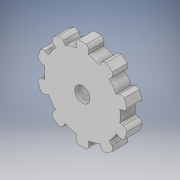
# Autodesk Inventor part: 10 ul Middle Gear
Saved by Autodesk Inventor 2017 (Build 210142000, 142)
## iProperties
Created: 2018-03-09
Part Number: 10 ul Middle Gear
Material: Generic
Document SubType Name: Modeling
Designer: Russ
Density: 1 g/cm^3
Appearance: Default
Author: Russ
Autodesk Inventor part; units mm, degrees
ref_plane "YZ Plane" through (0, 0, 0) normal (1, 0, 0) x (0, 1, 0)
ref_plane "XZ Plane" through (0, 0, 0) normal (0, 1, 0) x (-1, 0, 0)
ref_plane "XY Plane" through (0, 0, 0) normal (0, 0, 1) x (1, 0, 0)
sketch "Sketch1" plane through (0, 0, 0) normal (0, 0, 1) x (1, 0, 0)
  arc A0 (-1.49, 9.4077) -> (1.49, 9.4077) centre (0, 0) ccw
  line L0 (0, 9.525) -> (0, 11.43)
  line L1 (0, 11.43) -> (1.016, 11.43)
  line L2 (0, 11.43) -> (-1.016, 11.43)
  line L3 (-1.49, 9.4077) -> (-1.788, 11.2893)
  line L4 (-2.9434, 9.0588) -> (-3.5321, 10.8706)
  line L5 (-4.3243, 8.4868) -> (-5.1891, 10.1842)
  line L6 (-5.5987, 7.7059) -> (-6.7184, 9.2471)
  line L7 (-6.7352, 6.7352) -> (-8.0822, 8.0822)
  line L8 (-7.7059, 5.5987) -> (-9.2471, 6.7184)
  line L9 (-8.4868, 4.3243) -> (-10.1842, 5.1891)
  line L10 (-9.0588, 2.9434) -> (-10.8706, 3.5321)
  line L11 (-9.4077, 1.49) -> (-11.2893, 1.788)
  line L12 (-9.525, 0) -> (-11.43, 0)
  line L13 (-9.4077, -1.49) -> (-11.2893, -1.788)
  line L14 (-9.0588, -2.9434) -> (-10.8706, -3.5321)
  line L15 (-8.4868, -4.3243) -> (-10.1842, -5.1891)
  line L16 (-7.7059, -5.5987) -> (-9.2471, -6.7184)
  line L17 (-6.7352, -6.7352) -> (-8.0822, -8.0822)
  line L18 (-5.5987, -7.7059) -> (-6.7184, -9.2471)
  line L19 (-4.3243, -8.4868) -> (-5.1891, -10.1842)
  line L20 (-2.9434, -9.0588) -> (-3.5321, -10.8706)
  line L21 (-1.49, -9.4077) -> (-1.788, -11.2893)
  line L22 (0, -9.525) -> (0, -11.43)
  line L23 (1.49, -9.4077) -> (1.788, -11.2893)
  line L24 (2.9434, -9.0588) -> (3.5321, -10.8706)
  line L25 (4.3243, -8.4868) -> (5.1891, -10.1842)
  line L26 (5.5987, -7.7059) -> (6.7184, -9.2471)
  line L27 (6.7352, -6.7352) -> (8.0822, -8.0822)
  line L28 (7.7059, -5.5987) -> (9.2471, -6.7184)
  line L29 (8.4868, -4.3243) -> (10.1842, -5.1891)
  line L30 (9.0588, -2.9434) -> (10.8706, -3.5321)
  line L31 (9.4077, -1.49) -> (11.2893, -1.788)
  line L32 (9.525, 0) -> (11.43, 0)
  line L33 (9.4077, 1.49) -> (11.2893, 1.788)
  line L34 (9.0588, 2.9434) -> (10.8706, 3.5321)
  line L35 (8.4868, 4.3243) -> (10.1842, 5.1891)
  line L36 (7.7059, 5.5987) -> (9.2471, 6.7184)
  line L37 (6.7352, 6.7352) -> (8.0822, 8.0822)
  line L38 (5.5987, 7.7059) -> (6.7184, 9.2471)
  line L39 (4.3243, 8.4868) -> (5.1891, 10.1842)
  line L40 (2.9434, 9.0588) -> (3.5321, 10.8706)
  line L41 (1.49, 9.4077) -> (1.788, 11.2893)
  arc A1 (-1.016, 11.43) -> (-1.639, 10.3485) centre (-0.0747, 10.1675) ccw
  arc A2 (1.639, 10.3485) -> (1.016, 11.43) centre (0.0747, 10.1675) ccw
  dimension "d0" = 19.05
  dimension "d1" = 1.905
  dimension "d2" = 1.016
  dimension "d3" = 1.016
  dimension "d6" = 360
  dimension "d8" = 1.5748
  dimension "d9" = 1.5748
  constraints: 84 end point, 6 point on circle, 3 centre point, 2 horizontal, 2 midpoint, 1 coincident, 1 vertical, 121 other
  measures "d0" diameter of A0
  measures "d1" distance of L0.start L0.end
  measures "d2" distance of L0.end L1.end
  measures "d3" distance of L0.end L2.end
  measures "d8" radius of A1
  measures "d9" radius of A2
extrude "Extrusion1" add sketch "Sketch1" along normal blind 3.81
pattern_circular "Circular Pattern1" count 10 over 360 about axis through (0, 0, 0) along (0, 0, 1) of "Extrusion1"
sketch "Sketch2" plane through (0, 0, 3.81) normal (0, 0, 1) x (1, 0, 0)
  circle A0 centre (0, 0) radius 1.905
  dimension "d15" = 3.81
  constraints: 1 centre point, 1 coincident
  measures "d15" diameter of A0
extrude "Extrusion2" cut sketch "Sketch2" against normal up to next
body "Solid1"
